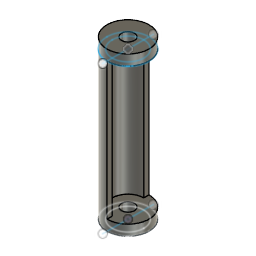
Support (Autodesk Fusion 360 design; units mm, degrees)
part number: 2026-06-24-14-55-54-877
Autodesk Fusion 360 part; units mm, degrees
note: some values were not read from the file. Set by a fixed rule: the direction of a hole.
sketch "Sketch1" plane through (0, 0, 0) normal (0, 0, 1) x (1, 0, 0)
  circle A0 centre (0, 0) radius 5
  circle A1 centre (0, 0) radius 3.75
  line L0 (0, 6) -> (0, -6)
  dimension "d1" = 10
  dimension "d10" = 7.5
  constraint coincident A0.centre A1.centre
  constraint concentric A0 A1
  constraint vertical L0
  measures "d1" diameter of A0
  measures "d10" diameter of A1
extrude "Extrude1" add sketch "Sketch1" along normal blind 2.5
extrude "Extrude2" add sketch "Sketch1" along normal blind 35 contours A0 A1 L0 picked at (-0.2484, 4.5647)
sketch "Sketch4" plane through (0, 0, 35) normal (0, 0, 1) x (-1, 0, 0)
  line L0 (0, -3.75) -> (0, -5)
  arc A0 (0, -5) -> (0, 5) centre (0, 0) ccw
  line L1 (0, 5) -> (0, 3.75)
  arc A1 (0, -3.75) -> (0, 3.75) centre (0, 0) ccw
  line L2 (0, 6) -> (0, -6)
  circle A2 centre (0, 0) radius 5
  circle A3 centre (0, 0) radius 3.75
  dimension "d13" = 10
  dimension "d14" = 7.5
  constraint coincident A0.centre A1.centre
  constraint concentric A2 A3
  constraint vertical L2
  measures "d13" diameter of A2
  measures "d14" diameter of A3
extrude "Extrude3" add sketch "Sketch4" along normal blind 2.5
hole "Hole3" at (0, 0, 35) direction (0, 0, 1) diameter 3.05 end through all
hole "Hole4" at (0, 0, 0) direction (0, 0, 1) diameter 3.05 end through all
